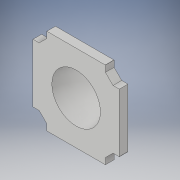
# Autodesk Inventor part: 20_Cube_Insert_Eye_v3
Saved by Autodesk Inventor 2019 (Build 230136000, 136)
## iProperties
Created: 2020-02-04
Part Number: 20_Cube_Insert_Eye_v3
Material: Generic
Document SubType Name: Modeling
Designer: marsikovabarbora
Density: 1 g/cm^3
Appearance: Default
Author: marsikovabarbora
Autodesk Inventor part; units mm, degrees
ref_plane "YZ Plane" through (0, 0, 0) normal (1, 0, 0) x (0, 1, 0)
ref_plane "XZ Plane" through (0, 0, 0) normal (0, 1, 0) x (-1, 0, 0)
ref_plane "XY Plane" through (0, 0, 0) normal (0, 0, 1) x (1, 0, 0)
sketch "Sketch1" plane through (0, 0, 0) normal (0, 0, 1) x (1, 0, 0)
  line L0 (-38.8739, 0) -> (58.9391, 0) construction
  line L1 (0, -36.2399) -> (0, 43.1348) construction
  line L2 (0, 0) -> (31.7956, 31.7956) construction
  line L3 (0, 0) -> (44.9658, 0) construction
  line L4 (0, 24.9006) -> (16.8, 24.9006)
  line L5 (16.8, 24.9006) -> (16.8, 21.2406)
  line L6 (16.8, 21.2406) -> (19.0203, 19.0203)
  line L7 (24.9006, 0) -> (24.9006, 16.8)
  line L8 (24.9006, 16.8) -> (21.2406, 16.8)
  line L9 (21.2406, 16.8) -> (19.0203, 19.0203)
  line L10 (0, 24.9006) -> (-16.8, 24.9006)
  line L11 (-16.8, 24.9006) -> (-16.8, 21.2406)
  line L12 (-16.8, 21.2406) -> (-19.0203, 19.0203)
  line L13 (-24.9006, 0) -> (-24.9006, 16.8)
  line L14 (-24.9006, 16.8) -> (-21.2406, 16.8)
  line L15 (-21.2406, 16.8) -> (-19.0203, 19.0203)
  line L16 (0, -24.9006) -> (16.8, -24.9006)
  line L17 (16.8, -24.9006) -> (16.8, -21.2406)
  line L18 (16.8, -21.2406) -> (19.0203, -19.0203)
  line L19 (24.9006, 0) -> (24.9006, -16.8)
  line L20 (24.9006, -16.8) -> (21.2406, -16.8)
  line L21 (21.2406, -16.8) -> (19.0203, -19.0203)
  line L22 (0, -24.9006) -> (-16.8, -24.9006)
  line L23 (-16.8, -24.9006) -> (-16.8, -21.2406)
  line L24 (-16.8, -21.2406) -> (-19.0203, -19.0203)
  line L25 (-24.9006, 0) -> (-24.9006, -16.8)
  line L26 (-24.9006, -16.8) -> (-21.2406, -16.8)
  line L27 (-21.2406, -16.8) -> (-19.0203, -19.0203)
  circle A0 centre (0, 0) radius 14
  dimension "d0" = 45
  dimension "d1" = 16.8
  dimension "d2" = 3.66
  dimension "d3" = 3.14
  dimension "d4" = 28
  constraints: 52 end point, 20 symmetric about line, 2 horizontal, 2 perpendicular, 2 point on line, 1 centre point, 1 coincident, 1 equal length
  measures "d0" angle of L3 L2
  measures "d1" distance of L4.start L4.end
  measures "d2" distance of L4.end L5.end
  measures "d3" distance of L5.end L6.end
  measures "d4" diameter of A0
extrude "Extrusion1" add sketch "Sketch1" along normal blind 5
sketch "Sketch2" plane through (0, 0, 5) normal (0, 0, 1) x (1, 0, 0)
  circle A0 centre (0, 0) radius 14 construction
  line L0 (16.8, 24.9006) -> (-16.8, 24.9006) construction
  line L1 (-16.8, 24.9006) -> (-16.8, 21.2406) construction
  line L2 (-16.8, 21.2406) -> (-21.2406, 16.8) construction
  line L3 (-21.2406, 16.8) -> (-24.9006, 16.8) construction
  line L4 (-24.9006, 16.8) -> (-24.9006, -16.8) construction
  line L5 (-24.9006, -16.8) -> (-21.2406, -16.8) construction
  line L6 (-21.2406, -16.8) -> (-16.8, -21.2406) construction
  line L7 (-16.8, -21.2406) -> (-16.8, -24.9006) construction
  line L8 (-16.8, -24.9006) -> (16.8, -24.9006) construction
  line L9 (16.8, -24.9006) -> (16.8, -21.2406) construction
  line L10 (16.8, -21.2406) -> (21.2406, -16.8) construction
  line L11 (21.2406, -16.8) -> (24.9006, -16.8) construction
  line L12 (24.9006, -16.8) -> (24.9006, 16.8) construction
  line L13 (24.9006, 16.8) -> (21.2406, 16.8) construction
  line L14 (21.2406, 16.8) -> (16.8, 21.2406) construction
  line L15 (16.8, 21.2406) -> (16.8, 24.9006) construction
  line L16 (-34.8609, 0) -> (34.8609, 0) construction
  line L17 (0, -34.8609) -> (0, 34.8609) construction
  circle A1 centre (13, -13) radius 2.5
  circle A2 centre (-13, -13) radius 2.5
  dimension "d7" = 5
  dimension "d8" = 13
  dimension "d9" = 13
  constraints: 2 centre point, 1 symmetric about line, 1 other
  measures "d7" diameter of A1
  measures "d8" distance from line of L16 A1.centre
  measures "d9" distance from line of L17 A1.centre
extrude "Extrusion2" [suppressed]
sketch "Sketch3" plane through (0, 0, 0) normal (1, 0, 0) x (0, 1, 0)
  line L0 (-14, 5) -> (14, 5) construction
  line L1 (24.9006, 5) -> (21.2406, 5) construction
  line L2 (21.2406, 5) -> (16.8, 5) construction
  line L3 (16.8, 5) -> (-16.8, 5) construction
  line L4 (-16.8, 5) -> (-21.2406, 5) construction
  line L5 (-21.2406, 5) -> (-24.9006, 5) construction
  line L6 (-24.9006, 5) -> (-21.2406, 5) construction
  line L7 (-21.2406, 5) -> (-16.8, 5) construction
  line L8 (-16.8, 5) -> (16.8, 5) construction
  line L9 (16.8, 5) -> (21.2406, 5) construction
  line L10 (21.2406, 5) -> (24.9006, 5) construction
  line L11 (24.9006, 0) -> (21.2406, 0) construction
  line L12 (24.9006, 0) -> (24.9006, 5) construction
  line L13 (21.2406, 5) -> (24.9006, 5) construction
  line L14 (21.2406, 0) -> (21.2406, 5) construction
  line L15 (21.2406, 0) -> (16.8, 0) construction
  line L16 (21.2406, 0) -> (21.2406, 5) construction
  line L17 (16.8, 5) -> (21.2406, 5) construction
  line L18 (16.8, 0) -> (16.8, 5) construction
  line L19 (16.8, 0) -> (-16.8, 0) construction
  line L20 (16.8, 0) -> (16.8, 5) construction
  line L21 (-16.8, 5) -> (16.8, 5) construction
  line L22 (-16.8, 0) -> (-16.8, 5) construction
  line L23 (-16.8, 0) -> (-21.2406, 0) construction
  line L24 (-16.8, 0) -> (-16.8, 5) construction
  line L25 (-21.2406, 5) -> (-16.8, 5) construction
  line L26 (-21.2406, 0) -> (-21.2406, 5) construction
  line L27 (-21.2406, 0) -> (-24.9006, 0) construction
  line L28 (-21.2406, 0) -> (-21.2406, 5) construction
  line L29 (-24.9006, 5) -> (-21.2406, 5) construction
  line L30 (-24.9006, 0) -> (-24.9006, 5) construction
  line L31 (-14, 5) -> (14, 5) construction
  line L32 (14, 0) -> (-14, 0) construction
  line L33 (16.8, 5) -> (-16.8, 5)
  arc A0 (0, -9) -> (14, 5) centre (0, 5) ccw
  line L34 (0, -16.0037) -> (0, 8.5006) construction
  arc A1 (0, -11) -> (16, 5) centre (0, 5) ccw
  line L35 (0, -9) -> (0, -11)
  line L36 (16, 5) -> (14, 5)
revolve "Revolution1" add sketch "Sketch3" angle 360 about axis through (0, 0, -10) along (0, 0, 1)
sketch "Skizze4" plane through (0, 0, 5) normal (0, 0, 1) x (1, 0, 0)
  circle A0 centre (0, 0) radius 14 construction
  line L0 (16.8, 24.9006) -> (-16.8, 24.9006) construction
  line L1 (-16.8, 24.9006) -> (-16.8, 21.2406) projected
  line L2 (-16.8, 21.2406) -> (-21.2406, 16.8) projected
  line L3 (-21.2406, 16.8) -> (-24.9006, 16.8) projected
  line L4 (-24.9006, 16.8) -> (-24.9006, -16.8) construction
  line L5 (-24.9006, -16.8) -> (-21.2406, -16.8) projected
  line L6 (-21.2406, -16.8) -> (-16.8, -21.2406) projected
  line L7 (-16.8, -21.2406) -> (-16.8, -24.9006) projected
  line L8 (-16.8, -24.9006) -> (16.8, -24.9006) construction
  line L9 (16.8, -24.9006) -> (16.8, -21.2406) projected
  line L10 (16.8, -21.2406) -> (21.2406, -16.8) projected
  line L11 (21.2406, -16.8) -> (24.9006, -16.8) projected
  line L12 (24.9006, -16.8) -> (24.9006, 16.8) construction
  line L13 (24.9006, 16.8) -> (21.2406, 16.8) projected
  line L14 (21.2406, 16.8) -> (16.8, 21.2406) projected
  line L15 (16.8, 21.2406) -> (16.8, 24.9006) projected
  line L16 (-16.9, 25.0006) -> (16.9, 25.0006) construction
  line L17 (16.9, 25.0006) -> (16.9, 21.2821)
  line L18 (16.9, 21.2821) -> (21.2821, 16.9)
  line L19 (21.2821, 16.9) -> (25.0006, 16.9)
  line L20 (25.0006, 16.9) -> (25.0006, -16.9) construction
  line L21 (25.0006, -16.9) -> (21.2821, -16.9)
  line L22 (21.2821, -16.9) -> (16.9, -21.2821)
  line L23 (16.9, -21.2821) -> (16.9, -25.0006)
  line L24 (16.9, -25.0006) -> (-16.9, -25.0006) construction
  line L25 (-16.9, -25.0006) -> (-16.9, -21.2821)
  line L26 (-16.9, -21.2821) -> (-21.2821, -16.9)
  line L27 (-21.2821, -16.9) -> (-25.0006, -16.9)
  line L28 (-25.0006, -16.9) -> (-25.0006, 16.9) construction
  line L29 (-25.0006, 16.9) -> (-21.2821, 16.9)
  line L30 (-21.2821, 16.9) -> (-16.9, 21.2821)
  line L31 (-16.9, 21.2821) -> (-16.9, 25.0006)
  line L32 (-24.9006, 16.8) -> (-24.9006, 16.9)
  line L33 (16.8, 24.9006) -> (-16.8, 24.9006) projected
  line L34 (-16.8, 24.9006) -> (-16.9, 24.9006)
  line L35 (16.8, 24.9006) -> (16.9, 24.9006)
  line L36 (24.9006, -16.8) -> (24.9006, 16.8) projected
  line L37 (24.9006, 16.8) -> (24.9006, 16.9)
  line L38 (24.9006, -16.8) -> (24.9006, -16.9)
  line L39 (16.8, -24.9006) -> (16.8, -21.2406) projected
  line L40 (16.8, -24.9006) -> (16.9, -24.9006)
  line L41 (-16.8, -24.9006) -> (-16.9, -24.9006)
  line L42 (-24.9006, -16.8) -> (-24.9006, 16.8) projected
  line L43 (-24.9006, -16.8) -> (-24.9006, -16.9)
  dimension "d15" = 0.1
  constraints: 48 end point, 12 point on line, 4 perpendicular, 15 other
  measures "d15" distance between parallel lines of L0 L16
extrude "IM_offset" add sketch "Skizze4" against normal up to surface (5 mm away)
equation "\"d9\" = d8"
body "Solid1"
